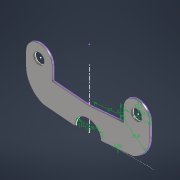
# Autodesk Inventor part: FixaçãoTanque_1
Saved by Autodesk Inventor 2022 (Build 260153000, 153)
## iProperties
Created: 2022-05-19
Part Number: FixaçãoTanque_1
Material: Liga de aço
Document SubType Name: Modeling
Designer: Gugarauj07
Density: 7.73 g/cm^3
Appearance: Semipolido
Author: Gugarauj07
Autodesk Inventor part; units mm, degrees
ref_plane "YZ Plane" through (0, 0, 0) normal (1, 0, 0) x (0, 1, 0)
ref_plane "XZ Plane" through (0, 0, 0) normal (0, 1, 0) x (-1, 0, 0)
ref_plane "XY Plane" through (0, 0, 0) normal (0, 0, 1) x (1, 0, 0)
sketch "Esboço1" plane through (0, 0, 0) normal (0, 0, 1) x (1, 0, 0)
  arc A0 (0, 12.7) -> (-12.7, 0) centre (0, 0) ccw
  circle A1 centre (-47.371, 39.2) radius 5.08
  line L0 (0, 0) -> (0, 58.6538)
  arc A2 (12.7, 0) -> (0, 12.7) centre (0, 0) ccw
  circle A3 centre (47.371, 39.2) radius 5.08
  line L1 (12.7, 0) -> (43.538, 2.698)
  line L2 (12.7, 0) -> (62.7, 0) construction
  arc A4 (60.071, 39.2) -> (34.671, 39.2) centre (47.371, 39.2) ccw
  line L3 (-12.7, 0) -> (-43.538, 2.698)
  arc A5 (-34.671, 39.2) -> (-60.071, 39.2) centre (-47.371, 39.2) ccw
  line L4 (34.671, 39.2) -> (34.671, 26.5)
  line L5 (-34.671, 39.2) -> (-34.671, 26.5)
  line L6 (60.071, 39.2) -> (60.071, 26.5)
  arc A6 (43.538, 2.698) -> (60.071, 26.5) centre (34.671, 26.5) ccw
  line L7 (-60.071, 39.2) -> (-60.071, 26.5)
  arc A7 (-60.071, 26.5) -> (-43.538, 2.698) centre (-34.671, 26.5) ccw
  line L8 (34.671, 26.5) -> (4.7852, 23.8853)
  line L9 (-34.671, 26.5) -> (-4.7852, 23.8853)
  arc A8 (-4.7852, 23.8853) -> (4.7852, 23.8853) centre (0, 74.0401) ccw
  point P0 (0, 25.2951)
  point P1 (0, 24.8739)
  dimension "d6" = 12.7
  dimension "d10" = 25.4
  dimension "d17" = 5
  dimension "d18" = 12.7
  dimension "d19" = 25.4
  dimension "d20" = 12.7
  dimension "d27" = 12.7
  dimension "d36" = 25.4
  dimension "d37" = 30
  constraints: 20 end point, 14 point on circle, 11 symmetric about line, 9 centre point, 3 vertical, 2 point on line, 1 coincident, 1 horizontal, 1 parallel, 9 other
  measures "d6" radius of A0
  measures "d10" distance of L1.start L3.start
  measures "d17" angle of L2 L1
  measures "d18" distance of A3.centre L6.start
  measures "d19" distance of L6.start L4.start
  measures "d20" radius of A4
  measures "d27" distance of L4.start L4.end
  measures "d36" radius of A6
  measures "d37" distance of L4.end L8.end
extrude "Extrusion2" add sketch "Esboço1" along normal blind 1.5
